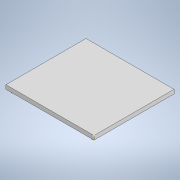
# Autodesk Inventor part: bottom part
Saved by Autodesk Inventor 2021 (Build 250183000, 183)
## iProperties
Created: 2021-07-07
Part Number: bottom part
Material: Generic
Document SubType Name: Modeling
Designer: VK
Density: 1 g/cm^3
Appearance: Default
Author: VK
Autodesk Inventor part; units mm, degrees
ref_plane "YZ Plane" through (0, 0, 0) normal (1, 0, 0) x (0, 1, 0)
ref_plane "XZ Plane" through (0, 0, 0) normal (0, 1, 0) x (-1, 0, 0)
ref_plane "XY Plane" through (0, 0, 0) normal (0, 0, 1) x (1, 0, 0)
sketch "Sketch1" plane through (0, 0, 0) normal (0, 1, 0) x (-1, 0, 0)
  line L0 (0, 0) -> (110, 0)
  line L1 (110, 0) -> (110, -100)
  line L2 (110, -100) -> (0, -100)
  line L3 (0, -100) -> (0, 0)
  dimension "d0" = 110
  dimension "d1" = 100
  constraints: 8 end point, 2 parallel, 1 horizontal, 1 perpendicular
  measures "d0" distance of L1.end L2.end
  measures "d1" distance of L0.end L1.end
extrude "Extrusion1" add sketch "Sketch1" along normal blind 5
sketch "Sketch2" plane through (0, 5, 0) normal (0, 1, 0) x (1, 0, 0)
  point P0 (0, 0)
sketch "Sketch3" plane through (0, 0, 0) normal (0, -1, 0) x (1, 0, 0)
  circle A0 centre (-4, -2.5) radius 1.5
  point P0 (0, 0)
  dimension "d4" = 3
  constraints: 1 centre point, 1 coincident
  measures "d4" diameter of A0
extrude "Extrusion2" add sketch "Sketch3" along normal blind 1.5
sketch "Sketch4" plane through (-4, -1.5, -2.5) normal (0, -1, 0) x (1, 0, 0)
  point P0 (4, 2.5)
sketch "Sketch5" plane through (-4, -1.5, -2.5) normal (0, -1, 0) x (1, 0, 0)
  line L0 (1.5, 0.5) -> (-1.5, 0.5)
  line L1 (-1.5, 0.5) -> (-1.5, -0.5)
  line L2 (-1.5, -0.5) -> (1.5, -0.5)
  line L3 (1.5, -0.5) -> (1.5, 0.5)
  line L4 (1.5, 0.5) -> (-1.5, -0.5) construction
  line L5 (-1.5, 0.5) -> (1.5, -0.5) construction
  point P0 (4, 2.5)
  point P1 (0, 0)
  dimension "d7" = 1
  constraints: 12 end point, 2 midpoint, 2 parallel, 1 horizontal, 1 perpendicular
  measures "d7" distance of L1.end L0.end
extrude "Extrusion3" cut sketch "Sketch5" against normal blind 1
pattern_linear "Rectangular Pattern1" count 2 spacing 100 along (-1, 0, 0) of "Extrusion3", "Extrusion2"
pattern_linear "Rectangular Pattern2" count 2 spacing 95 along (0, 0, -1) of "Extrusion2", "Extrusion3"
pattern_linear "Rectangular Pattern3" count 2 spacing 95 along (0, 0, -1) of "Extrusion3", "Extrusion2", "Rectangular Pattern1"
body "Solid1"
